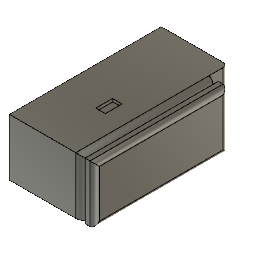
Mary project v1 (Autodesk Fusion 360 design; units mm, degrees)
Autodesk Fusion 360 part; units mm, degrees
sketch "Sketch1" plane through (0, 0, 0) normal (0, 0, 1) x (1, 0, 0)
  line L0 (40, -70) -> (-40, -70)
  line L1 (-40, -70) -> (-40, 70)
  line L2 (-40, 70) -> (40, 70)
  line L3 (40, 70) -> (40, -70)
  line L4 (40, -70) -> (-40, 70) construction
  line L5 (-40, -70) -> (40, 70) construction
  constraint horizontal L0
  constraint perpendicular L0 L1
  constraint parallel L0 L2
  constraint parallel L1 L3
  constraint coincident L4 origin
  constraint coincident L5 origin
extrude "Extrude1" add sketch "Sketch1" along normal blind 60
sketch "Sketch2" plane through (40, 0, 0) normal (1, 0, 0) x (0, 1, 0)
  line L0 (-70, 0) -> (70, 0)
  line L1 (70, 0) -> (70, 60)
  line L2 (70, 60) -> (-70, 60)
  line L3 (-70, 60) -> (-70, 0)
fillet "Fillet1" radius 10 3 edges at (40, 0, 60) (40, -70, 30) (40, 70, 30)
extrude "Extrude2" add sketch "Sketch2" along normal blind 10
extrude "Extrude3" add 1 faces at (-16.6667, 70, 20) along direction (0, 1, 0) blind 20
sketch "Sketch3" plane through (0, 0, 0) normal (1, 0, 0) x (0, 1, 0)
  line L0 (-1.1501, 56.847) -> (-18.8499, 56.847)
  line L1 (-18.8499, 56.847) -> (-18.8499, 63.153)
  line L2 (-18.8499, 63.153) -> (-1.1501, 63.153)
  line L3 (-1.1501, 63.153) -> (-1.1501, 56.847)
  line L4 (-1.1501, 56.847) -> (-18.8499, 63.153) construction
  line L5 (-18.8499, 56.847) -> (-1.1501, 63.153) construction
  point P0 (-10, 60)
  constraint horizontal L0
  constraint perpendicular L0 L1
  constraint parallel L0 L2
  constraint parallel L1 L3
  constraint coincident L4 P0
  constraint coincident L5 P0
extrude "Extrude4" cut sketch "Sketch3" along normal blind 10
fillet "Fillet2" radius 5 1 edges at (50, 0, 60) 1 faces at (50, -23.3333, 40)
sketch "Sketch4" plane through (0, 0, 0) normal (1, 0, 0) x (0, 1, 0)
  line L0 (7.722, -4.2717) -> (-7.722, -4.2717)
  line L1 (-7.722, -4.2717) -> (-7.722, 4.2717)
  line L2 (-7.722, 4.2717) -> (7.722, 4.2717)
  line L3 (7.722, 4.2717) -> (7.722, -4.2717)
  line L4 (7.722, -4.2717) -> (-7.722, 4.2717) construction
  line L5 (-7.722, -4.2717) -> (7.722, 4.2717) construction
  constraint horizontal L0
  constraint perpendicular L0 L1
  constraint parallel L0 L2
  constraint parallel L1 L3
  constraint coincident L4 origin
  constraint coincident L5 origin
extrude "Extrude5" cut sketch "Sketch4" along normal blind 5
fillet "Fillet3" radius 5 1 edges at (30, 90, 30)
